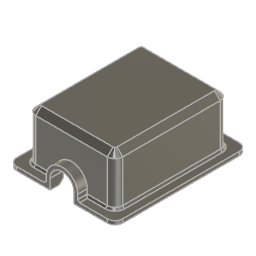
Freezer Door Switch Wiring Cover (Autodesk Fusion 360 design; units mm, degrees)
Autodesk Fusion 360 part; units mm, degrees
sketch "Sketch1" plane through (0, 0, 0) normal (0, 0, 1) x (1, 0, 0)
  line L0 (-27.7, 69) -> (27.7, 69)
  line L1 (27.7, 69) -> (27.7, 0)
  line L2 (27.7, 0) -> (-27.7, 0)
  line L3 (-27.7, 0) -> (-27.7, 69)
  line L4 (22.7, 64) -> (22.7, 5)
  line L5 (22.7, 5) -> (-22.7, 5)
  line L6 (-22.7, 5) -> (-22.7, 64)
  line L7 (-22.7, 64) -> (22.7, 64)
  line L8 (0, 0) -> (0, 5) construction
  line L9 (-8.2, 5) -> (-8.2, 0)
  line L10 (8.2, 5) -> (8.2, 0)
  dimension "d1" = 55.4
  dimension "d2" = 69
  dimension "d3" = 5
  dimension "d4" = 16.4
  constraint horizontal L0
  constraint vertical L1
  constraint horizontal L2
  constraint vertical L3
  constraint midpoint L2 L8.start
  constraint coincident L8.start origin
  constraint midpoint L5 L8.end
  constraint coincident L5 L9.start
  constraint coincident L2 L9.end
  constraint perpendicular L2 L9
  constraint symmetric L8 L9.start L10.start
  constraint symmetric L8 L9.end L10.end
  measures "d1" distance of L1.end L2.end
  measures "d2" distance of L0.end L1.end
  measures "d4" distance of L9 L10
extrude "Extrude1" add sketch "Sketch1" along normal blind 28 contours L4 L5 L6 L7
extrude "Extrude2" add sketch "Sketch1" along normal blind 2 contours L0 L1 L2 L3 L4 L5 L6 L7 L9 L10 | L2 L5 L9 L10
fillet "Fillet1" radius 4 8 edges at (-27.7, 0, 1) (27.7, 0, 1) (22.7, 5, 15) (-22.7, 5, 15) (-27.7, 69, 1) (-22.7, 64, 15) (27.7, 69, 1) (22.7, 64, 15)
chamfer "Chamfer1" distance 3 angle 45 8 edges at (22.7, 34.5, 28) (21.5284, 62.8284, 28) (0, 64, 28) (-21.5284, 62.8284, 28) (-22.7, 34.5, 28) (-21.5284, 6.1716, 28) (0, 5, 28) (21.5284, 6.1716, 28)
chamfer "Chamfer2" distance 1 angle 45 8 edges at (22.7, 34.5, 2) (21.5284, 62.8284, 2) (0, 64, 2) (-21.5284, 62.8284, 2) (-22.7, 34.5, 2) (-21.5284, 6.1716, 2) (0, 5, 2) (21.5284, 6.1716, 2)
shell "Shell1" thickness 2 removed faces 1 at (-9.2333, 44.6667, 0)
sketch "Sketch2" plane through (0, 0, 0) normal (0, -1, 0) x (1, 0, 0)
  line L0 (23.7, 0) -> (23.7, 2)
  line L1 (23.7, 2) -> (-23.7, 2)
  line L2 (-23.7, 2) -> (-23.7, 0)
  line L3 (-23.7, 0) -> (23.7, 0)
  line L4 (-8.2, 0) -> (-8.2, 5.4)
  line L5 (8.2, 0) -> (8.2, 5.4)
  arc A0 (8.2, 5.4) -> (-8.2, 5.4) centre (0, 5.4) ccw
  line L6 (-6.2, 0) -> (-6.2, 5.4)
  arc A1 (6.2, 5.4) -> (-6.2, 5.4) centre (0, 5.4) ccw
  line L7 (6.2, 0) -> (6.2, 5.4)
  line L8 (-8.2, 0) -> (-6.2, 0)
  line L9 (6.2, 0) -> (8.2, 0)
  line L10 (-6.2, 0) -> (6.2, 0)
  point P0 (-8.2, 0)
  point P1 (8.2, 0)
  dimension "d14" = 2
  dimension "d15" = 11.6
  constraint coincident P0 L4.start
  constraint perpendicular L1 L4
  constraint coincident P1 L5.start
  constraint perpendicular L3 L5
  constraint equal L4 L5
  constraint tangent L4 A0
  constraint perpendicular L6 L8
  constraint perpendicular L7 L9
extrude "Extrude3" add sketch "Sketch2" against normal up to surface (5 mm away) contours L1 L4 L5 A0 L6 A1 L7
extrude "Extrude4" cut sketch "Sketch2" against normal up to surface (7 mm away) contours L1 L3 L6 L7 L10 | L1 L6 A1 L7
chamfer "Chamfer3" distance 1 angle 45 2 edges at (-8.2, 2, 2) (8.2, 2, 2)
named bodies: "Freezer Door Switch Cover"
